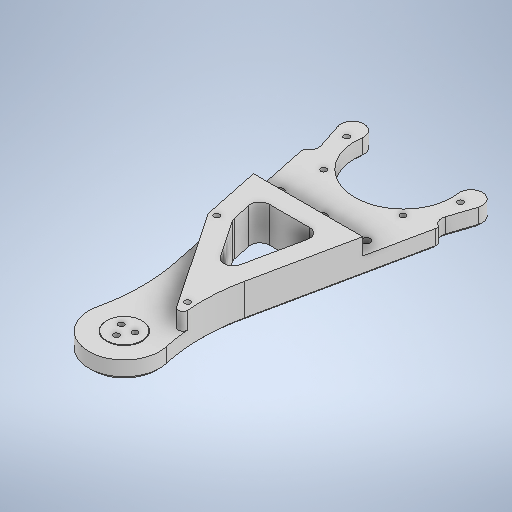
# Autodesk Inventor part: motion_thigh_top_R
Saved by Autodesk Inventor 2025.2 (Build 292293000, 293)
## iProperties
Created: 2025-04-10
Part Number: motion_thigh_top_R
Material: Generic
Document SubType Name: Modeling
Designer: Bruno
Density: 1 g/cm^3
Appearance: Default
Mass: 96.8952 g
Surface Area: 228.709 cm^2
Volume: 96.8952 cm^3
Author: Bruno
## iProperties of the stored document motion_thigh_top_R_3DPrint.ipt
Created: 2025-04-29
Part Number: motion_thigh_top_R_3DPrint
Material: Generic
Document SubType Name: Modeling
Designer: Bruno
Density: 1 g/cm^3
Appearance: Default
Author: Bruno
Autodesk Inventor part; units mm, degrees
ref_plane "YZ Plane" through (0, 0, 0) normal (1, 0, 0) x (0, 1, 0)
ref_plane "XZ Plane" through (0, 0, 0) normal (0, 1, 0) x (-1, 0, 0)
ref_plane "XY Plane" through (0, 0, 0) normal (0, 0, 1) x (1, 0, 0)
sketch "Sketch1" plane through (0, 0, 0) normal (0, 1, 0) x (-1, 0, 0)
  line L0 (0, -140.06) -> (0, 133.01) construction
  line L1 (42.5247, -92.2999) -> (20, -23.7432)
  line L2 (20, -23.7432) -> (-20, -23.7432) construction
  line L3 (-20, -23.7432) -> (-42.5247, -92.2999)
  circle A0 centre (30.55, -75) radius 1.5
  circle A1 centre (21.275, -53.4355) radius 1.5
  circle A2 centre (12, -31.8711) radius 2
  circle A3 centre (0, -31.8711) radius 2
  circle A4 centre (-12, -31.8711) radius 2
  circle A5 centre (-21.275, -53.4355) radius 1.5
  circle A6 centre (-30.55, -75) radius 1.5
  circle A7 centre (0, -75) radius 26.05
  line L4 (0, -75) -> (0, 75) construction
  arc A8 (18.259, 69.7455) -> (-18.259, 69.7455) centre (0, 75) ccw
  arc A9 (18.259, 69.7455) -> (20, -23.7432) centre (170.8734, 25.8271) ccw
  arc A10 (-20, -23.7432) -> (-18.259, 69.7455) centre (-170.8734, 25.8271) ccw
  circle A11 centre (31.8586, -79.425) radius 6.1144
  circle A12 centre (-31.8586, -79.425) radius 6.1144
  point P0 (0, 0)
  point P1 (37.6675, -77.5164)
  point P2 (-37.6675, -77.5164)
  point P3 (-25.8023, -78.5838)
  point P4 (25.8023, -78.5838)
  dimension "d0" = 3
  dimension "d1" = 52.1
  dimension "d2" = 4
  dimension "d3" = 36.376
  dimension "d4" = 108.188
  dimension "d5" = 80.8
  dimension "d6" = 68.5567
  dimension "d7" = 80.8
  dimension "d8" = 5.9764
  dimension "d9" = 64.0236
  dimension "d10" = 35
  dimension "d11" = 35
  dimension "d12" = 64.0236
  dimension "d13" = 5.9764
  dimension "d14" = 8.0569
  dimension "d15" = 48.4809
  dimension "d16" = 48.4809
  dimension "d17" = 8.0569
  dimension "d18" = 10.1373
  dimension "d19" = 32.9382
  dimension "d20" = 21.5378
  dimension "d21" = 21.5378
  dimension "d22" = 32.9382
  dimension "d23" = 10.1373
  dimension "d24" = 150
  dimension "d25" = 38
  dimension "d26" = 75
  constraints: 13 centre point, 10 tangent, 8 end point, 6 point on circle, 5 equal radius, 2 point on line, 2 vertical alignment, 1 coincident
  measures "d0" diameter of A0
  measures "d1" diameter of A7
  measures "d2" diameter of A2
  measures "d3" angle of L1 L3
  measures "d4" angle of L1 L2
  measures "d5" distance from line of L1.start L3
  measures "d6" distance from line of L1.start L2
  measures "d7" distance from line of L3.end L1
  measures "d8" distance from line of A0.centre L1
  measures "d9" distance from line of A0.centre L3
  measures "d10" distance from line of L4.start L1
  measures "d11" distance from line of L4.start L3
  measures "d12" distance from line of A6.centre L1
  measures "d13" distance from line of A6.centre L3
  measures "d14" distance from line of A1.centre L1
  measures "d15" distance from line of A1.centre L3
  measures "d16" distance from line of A5.centre L1
  measures "d17" distance from line of A5.centre L3
  measures "d18" distance from line of A2.centre L1
  measures "d19" distance from line of A2.centre L3
  measures "d20" distance from line of A3.centre L1
  measures "d21" distance from line of A3.centre L3
  measures "d22" distance from line of A4.centre L1
  measures "d23" distance from line of A4.centre L3
  measures "d24" distance of L4.start L4.end
  measures "d25" diameter of A8
  measures "d26" distance of point (0, 0) L4.end
extrude "Extrusion1" add sketch "Sketch1" along normal blind 10 contours A11 A7 A12 L3 A10 A8 A9 L1 | A11 | A12 | A2 | A4
sketch "Sketch2" plane through (0, 0, 0) normal (0, -1, 0) x (1, 0, 0)
  arc A0 (18.259, 69.7455) -> (20, -23.7432) centre (170.8734, 25.8271) ccw projected
  line L0 (20, -23.7432) -> (-20, -23.7432)
  arc A1 (18.259, 69.7455) -> (-18.259, 69.7455) centre (0, 75) ccw projected
  arc A2 (-20, -23.7432) -> (-18.259, 69.7455) centre (-170.8734, 25.8271) ccw projected
  circle A3 centre (0, 75) radius 24 construction
  arc A4 (-8.448, 56.1313) -> (-14.4134, 53.0348) centre (-10.9405, 53.6387) ccw
  arc A5 (12.2645, 33.7778) -> (11.2365, 36.4468) centre (8.7439, 33.9542) ccw
  line L1 (-8.448, 56.1313) -> (11.2365, 36.4468)
  line L2 (0, 75) -> (0, 70.3396) construction
  point P0 (0, 0)
  dimension "d30" = 48
  dimension "d31" = 7.05
  dimension "d32" = 7.05
  dimension "d33" = 45
  constraints: 6 end point, 6 point on circle, 4 tangent, 2 centre point, 1 coincident, 1 vertical, 3 other
  measures "d31" diameter of A4
  measures "d32" diameter of A5
  measures "d33" angle of L1 L2
sketch "Sketch4" plane through (0, 10, 0) normal (0, 1, 0) x (1, 0, 0)
  arc A0 (-18.259, -69.7455) -> (18.259, -69.7455) centre (0, -75) ccw projected
  circle A1 centre (0, -75) radius 8.5 construction
  line L0 (-3.6806, -70.075) -> (3.6806, -70.075) construction
  line L1 (2.4249, -80.65) -> (6.1055, -74.275) construction
  line L2 (-2.4249, -80.65) -> (-6.1055, -74.275) construction
  circle A2 centre (0, -75) radius 4.25 construction
  arc A3 (-2.7639, -79.6984) -> (2.7639, -79.6984) centre (0, -79.25) ccw
  arc A4 (5.4509, -75.0444) -> (2.687, -70.2572) centre (3.6806, -72.875) ccw
  arc A5 (-2.687, -70.2572) -> (-5.4509, -75.0444) centre (-3.6806, -72.875) ccw
  arc A6 (-2.687, -70.2572) -> (2.687, -70.2572) centre (0, -63.1778) ccw
  arc A7 (-2.7639, -79.6984) -> (-5.4509, -75.0444) centre (-10.2383, -80.9111) ccw
  arc A8 (5.4509, -75.0444) -> (2.7639, -79.6984) centre (10.2383, -80.9111) ccw
  point P0 (0, 0)
  dimension "d40" = 17
  dimension "d46" = 2.8
  dimension "d47" = 2.8
  dimension "d48" = 2.8
  dimension "d50" = 8.5
  constraints: 21 point on circle, 13 tangent, 8 centre point, 6 end point, 2 coincident, 2 equal length, 2 equal radius, 1 horizontal
  measures "d40" diameter of A1
  measures "d46" radius of A5
  measures "d47" radius of A4
  measures "d48" radius of A3
  measures "d50" diameter of A2
extrude "Extrusion4" cut sketch "Sketch4" against normal blind 3
sketch "Sketch5" plane through (0, 7, 0) normal (0, 1, 0) x (1, 0, 0)
  arc A0 (-2.687, -70.2572) -> (-5.4509, -75.0444) centre (-3.6806, -72.875) ccw projected
  circle A1 centre (-3.6806, -72.875) radius 1.5
  arc A2 (5.4509, -75.0444) -> (2.687, -70.2572) centre (3.6806, -72.875) ccw projected
  circle A3 centre (3.6806, -72.875) radius 1.5
  arc A4 (-2.7639, -79.6984) -> (2.7639, -79.6984) centre (0, -79.25) ccw projected
  circle A5 centre (0, -79.25) radius 1.5
  point P0 (0, 0)
  point P1 (-6.1055, -74.275)
  point P2 (-3.6806, -70.075)
  point P3 (3.6806, -70.075)
  point P4 (6.1055, -74.275)
  point P5 (2.4249, -80.65)
  point P6 (-2.4249, -80.65)
  dimension "d53" = 3
  dimension "d54" = 3
  dimension "d55" = 3
  constraints: 3 centre point, 3 coincident
  measures "d53" diameter of A1
  measures "d54" diameter of A5
  measures "d55" diameter of A3
extrude "Extrusion5" cut sketch "Sketch5" against normal through all
sketch "Sketch10" plane through (0, 10, 0) normal (0, 1, 0) x (1, 0, 0)
  point P0 (0, 0)
sketch "Sketch11" plane through (0, 10, 0) normal (0, 1, 0) x (1, 0, 0)
  circle A0 centre (23.2705, 31.8711) radius 2 projected
  circle A1 centre (-23.2705, 31.8711) radius 2 projected
  arc A2 (36.124, 56.2492) -> (35.2621, 58.3316) centre (34.1663, 56.6585) ccw projected
  arc A3 (33.2513, 64.0751) -> (35.2621, 58.3316) centre (38.0015, 62.5144) ccw projected
  line L0 (33.2513, 64.0751) -> (42.5247, 92.2999) projected
  arc A4 (37.4868, 95.4546) -> (42.5247, 92.2999) centre (43.0738, 98.7767) ccw projected
  line L1 (13.5182, 103.3296) -> (37.4868, 95.4546) projected
  line L2 (13.5182, 103.3296) -> (21.946, 128.9806) projected
  line L3 (44.7468, 121.4892) -> (21.946, 128.9806) projected
  line L4 (44.7468, 121.4892) -> (45.9436, 125.1317) projected
  arc A5 (45.9436, 125.1317) -> (-45.9436, 125.1317) centre (0, 75) ccw projected
  line L5 (-45.9436, 125.1317) -> (-41.8595, 112.7014) projected
  line L6 (-41.8595, 112.7014) -> (-19.0587, 120.1928) projected
  line L7 (-19.0587, 120.1928) -> (-16.4055, 112.1174) projected
  line L8 (-16.4055, 112.1174) -> (-39.2064, 104.6261) projected
  line L9 (-39.2064, 104.6261) -> (-38.9298, 103.7845) projected
  arc A6 (-42.5247, 92.2999) -> (-38.9298, 103.7845) centre (-43.0738, 98.7767) ccw projected
  line L10 (-42.5247, 92.2999) -> (-33.2513, 64.0751) projected
  arc A7 (-35.2621, 58.3316) -> (-33.2513, 64.0751) centre (-38.0015, 62.5144) ccw projected
  arc A8 (-35.2621, 58.3316) -> (-36.124, 56.2492) centre (-34.1663, 56.6585) ccw projected
  line L11 (-36.124, 56.2492) -> (-29.328, 23.7432) projected
  line L12 (-29.328, 23.7432) -> (29.328, 23.7432) projected
  line L13 (29.328, 23.7432) -> (36.124, 56.2492) projected
  circle A9 centre (-30.55, 75) radius 1.5 projected
  circle A10 centre (0, 31.8711) radius 2 projected
  circle A11 centre (30.55, 75) radius 1.5 projected
  circle A12 centre (-21.275, 53.4355) radius 1.5 projected
  circle A13 centre (21.275, 53.4355) radius 1.5 projected
  circle A14 centre (0, 75) radius 26.05 projected
  line L14 (-8.6089, 110.8133) -> (-15.4999, 131.7869) projected
  arc A15 (-14.0608, 134.3573) -> (-15.4999, 131.7869) centre (-13.5998, 132.4112) ccw projected
  arc A16 (14.0608, 134.3573) -> (-14.0608, 134.3573) centre (0, 75) ccw projected
  arc A17 (15.4999, 131.7869) -> (14.0608, 134.3573) centre (13.5998, 132.4112) ccw projected
  line L15 (15.4999, 131.7869) -> (8.6089, 110.8133) projected
  arc A18 (6.3466, 109.4706) -> (8.6089, 110.8133) centre (6.7088, 111.4375) ccw projected
  arc A19 (6.3466, 109.4706) -> (-6.3466, 109.4706) centre (0, 75) ccw projected
  arc A20 (-8.6089, 110.8133) -> (-6.3466, 109.4706) centre (-6.7088, 111.4375) ccw projected
  line L16 (20, 23.7432) -> (37.6675, 77.5164) projected
  line L17 (-37.6675, 77.5164) -> (-20, 23.7432) projected
  point P0 (0, 0)
  point P1 (22.1305, 30.2277)
  point P2 (23.3273, 33.8703)
  point P3 (-23.3273, 33.8703)
  point P4 (-22.1305, 30.2277)
extrude "Extrusion8" add sketch "Sketch11" against normal up to surface (10 mm away) contours A0 L16 | A0 L16 A3 A2 L13 L12 | L16 A0 | L12 L11 A8 A7 L17 A1 | L17 A1 | A1 L17
sketch "Sketch12" plane through (0, 10, 0) normal (0, 1, 0) x (1, 0, 0)
  circle A0 centre (-23.2705, 31.8711) radius 2 projected
  circle A1 centre (23.2705, 31.8711) radius 2 projected
  point P0 (0, 0)
extrude "Extrusion9" cut sketch "Sketch12" against normal through all
sketch "Sketch13" plane through (0, 10, 0) normal (0, 1, 0) x (1, 0, 0)
  line L0 (-36.124, 56.2492) -> (-29.328, 23.7432) projected
  line L1 (-29.328, 23.7432) -> (-18.3221, -28.899)
  arc A0 (-18.259, -69.7455) -> (18.259, -69.7455) centre (0, -75) ccw projected
  circle A1 centre (0, -75) radius 19
  arc A2 (-18.5539, -70.9068) -> (-18.3221, -28.899) centre (-116.2057, -49.3635) ccw
  line L2 (0, -56) -> (0, -94) construction
  line L3 (29.328, 23.7432) -> (18.3221, -28.899)
  arc A3 (18.3221, -28.899) -> (18.5539, -70.9068) centre (116.2057, -49.3635) ccw
  arc A4 (-18.259, -69.7455) -> (-20, 23.7432) centre (-170.8734, -25.8271) ccw projected
  line L4 (-29.328, 23.7432) -> (-20, 23.7432) projected
  line L5 (20, 23.7432) -> (29.328, 23.7432) projected
  arc A5 (20, 23.7432) -> (18.259, -69.7455) centre (170.8734, -25.8271) ccw projected
  point P0 (0, 0)
  point P1 (0, -75)
  point P2 (18.5539, -70.9068)
  point P3 (-18.5539, -70.9068)
  dimension "d67" = 100
  constraints: 8 point on circle, 6 end point, 4 symmetric about line, 3 centre point, 2 tangent, 1 coincident, 1 collinear, 1 concentric, 1 midpoint, 1 vertical alignment, 1 other
  measures "d67" radius of A2
extrude "Extrusion10" add sketch "Sketch13" against normal up to surface (10 mm away) contours L4 A4 A0 A2 L1 | A5 L5 L3 A3 A0
chamfer "Chamfer1" distance 2 angle 45 14 edges at (-27.2231, 10, -13.6751) (-16.2072, 10, 49.9152) (0, 10, 94) (16.2072, 10, 49.9152) (27.2231, 10, -13.6751) (36.0143, 10, -57.4234) (33.2823, 10, -60.8622) (35.4594, 10, -70.7958) (32.4064, 10, -85.5148) (0, 10, -48.95) (-32.4064, 10, -85.5148) (-35.4594, 10, -70.7958) (-33.2823, 10, -60.8622) (-36.0143, 10, -57.4234)
sketch "Sketch24" plane through (0, 0, 0) normal (0, -1, 0) x (1, 0, 0)
  line L0 (4.2583, 47.3257) -> (-95.4066, -100.5193) projected
  line L1 (-29.328, -23.7432) -> (29.328, -23.7432) projected
  arc A0 (18.5539, 70.9068) -> (18.3221, 28.899) centre (116.2057, 49.3635) ccw projected
  circle A1 centre (-23.2705, -31.8711) radius 2 projected
  circle A2 centre (23.2705, -31.8711) radius 2 projected
  arc A3 (18.5539, 70.9068) -> (-18.5539, 70.9068) centre (0, 75) ccw projected
  arc A4 (-18.3221, 28.899) -> (-18.5539, 70.9068) centre (-116.2057, 49.3635) ccw projected
  line L2 (-18.3221, 28.899) -> (-36.124, -56.2492) projected
  arc A5 (-36.124, -56.2492) -> (-35.2621, -58.3316) centre (-34.1663, -56.6585) ccw projected
  arc A6 (-33.2513, -64.0751) -> (-35.2621, -58.3316) centre (-38.0015, -62.5144) ccw projected
  line L3 (-37.6675, -77.5164) -> (-33.2513, -64.0751) projected
  arc A7 (-37.6675, -77.5164) -> (-25.8023, -78.5838) centre (-31.8586, -79.425) ccw projected
  arc A8 (25.8023, -78.5838) -> (-25.8023, -78.5838) centre (0, -75) ccw projected
  arc A9 (25.8023, -78.5838) -> (37.6675, -77.5164) centre (31.8586, -79.425) ccw projected
  line L4 (33.2513, -64.0751) -> (37.6675, -77.5164) projected
  arc A10 (35.2621, -58.3316) -> (33.2513, -64.0751) centre (38.0015, -62.5144) ccw projected
  arc A11 (35.2621, -58.3316) -> (36.124, -56.2492) centre (34.1663, -56.6585) ccw projected
  line L5 (36.124, -56.2492) -> (18.3221, 28.899) projected
  arc A12 (18.5539, 70.9068) -> (18.3221, 28.899) centre (116.2057, 49.3635) ccw projected
  circle A13 centre (3.6806, 72.875) radius 1.5 projected
  circle A14 centre (0, 79.25) radius 1.5 projected
  circle A15 centre (-3.6806, 72.875) radius 1.5 projected
  circle A16 centre (-30.55, -75) radius 1.5 projected
  circle A17 centre (30.55, -75) radius 1.5 projected
  circle A18 centre (0, -31.8711) radius 2 projected
  circle A19 centre (21.275, -53.4355) radius 1.5 projected
  circle A20 centre (-21.275, -53.4355) radius 1.5 projected
  line L6 (4.2583, 47.3257) -> (17.8664, 67.5123)
  point P0 (0, 0)
  point P1 (-22.8891, 7.0548)
  point P2 (18.3221, 28.899)
  constraints: 2 end point, 1 collinear, 1 point on circle
extrude "Extrusion20" add sketch "Sketch24" along normal blind 9 contours L6 A0 L5 L1 L2 L0
sketch "Sketch25" plane through (0, -9, 0) normal (0, -1, 0) x (1, 0, 0)
  circle A0 centre (13.8445, 83.053) radius 1.5 projected
  circle A1 centre (-8.053, 88.8445) radius 1.5 projected
  circle A2 centre (8.053, 61.1555) radius 1.5 projected
  circle A3 centre (-13.8445, 66.947) radius 1.5 projected
  circle A4 centre (57.0388, 59.9143) radius 1.5 projected
  circle A5 centre (0, 75) radius 12.1825 projected
  line L0 (54.7376, 51.2135) -> (22.5353, 59.7304) projected
  arc A6 (54.7376, 51.2135) -> (59.34, 68.6151) centre (57.0388, 59.9143) ccw projected
  line L1 (27.1377, 77.132) -> (59.34, 68.6151) projected
  arc A7 (15.9979, 85.2502) -> (27.1377, 77.132) centre (31.9958, 95.5005) ccw projected
  arc A8 (15.9979, 85.2502) -> (8.8386, 58.181) centre (0, 75) ccw projected
  arc A9 (22.5353, 59.7304) -> (8.8386, 58.181) centre (17.6772, 41.362) ccw projected
  line L2 (17.8664, 67.5123) -> (-22.8891, 7.0548) projected
  line L3 (-22.8891, 7.0548) -> (-29.328, -23.7432) projected
  line L4 (-29.328, -23.7432) -> (29.328, -23.7432) projected
  line L5 (29.328, -23.7432) -> (18.3221, 28.899) projected
  arc A10 (17.8664, 67.5123) -> (18.3221, 28.899) centre (116.2057, 49.3635) ccw projected
  circle A11 centre (14.0822, 57.5183) radius 2.4486
  arc A12 (17.8664, 67.5123) -> (18.3221, 28.899) centre (116.2057, 49.3635) ccw projected
  arc A13 (-22.5029, 7.6276) -> (-23.0304, 6.3786) centre (-19.58, 5.6572) ccw
  point P0 (0, 0)
  point P1 (16.523, 57.3234)
  point P2 (12.0519, 58.8869)
  dimension "d117" = 7.05
  constraints: 5 tangent, 2 centre point, 2 point on circle, 2 point on line
  measures "d117" diameter of A13
extrude "Extrusion21" cut sketch "Sketch25" against normal up to surface (9 mm away) contours A10 A11 A9 | A9 L2 A10 | A11 L2 A9 | A13 L3 L2
sketch "Sketch26" plane through (0, -9, 0) normal (0, -1, 0) x (1, 0, 0)
  circle A0 centre (12.7693, 53.6449) radius 3.525 construction
  arc A1 (16.523, 57.3234) -> (18.3221, 28.899) centre (116.2057, 49.3635) ccw projected
  line L0 (12.0519, 58.8869) -> (-22.5029, 7.6276) projected
  circle A2 centre (12.7693, 53.6449) radius 1.5
  arc A3 (-22.5029, 7.6276) -> (-23.0304, 6.3786) centre (-19.58, 5.6572) ccw projected
  circle A4 centre (-19.58, 5.6572) radius 1.5
  point P0 (0, 0)
  dimension "d120" = 7.05
  dimension "d121" = 3
  dimension "d122" = 3
  constraints: 3 centre point, 2 coincident, 2 tangent
  measures "d120" diameter of A0
  measures "d121" diameter of A2
  measures "d122" diameter of A4
extrude "Extrusion22" cut sketch "Sketch26" against normal through all
sketch "Sketch27" plane through (0, 10, 0) normal (0, 1, 0) x (1, 0, 0)
  circle A0 centre (-19.58, -5.6572) radius 1.5 projected
  circle A1 centre (-19.58, -5.6572) radius 2.8
  circle A2 centre (12.7693, -53.6449) radius 1.5 projected
  circle A3 centre (12.7693, -53.6449) radius 2.8
  point P0 (0, 0)
  dimension "d125" = 5.6
  dimension "d126" = 5.6
  constraints: 2 centre point, 2 coincident
  measures "d125" diameter of A1
  measures "d126" diameter of A3
extrude "Extrusion23" cut sketch "Sketch27" against normal blind 3 contours A0 | A1 | A2 | A3
sketch "Sketch28" plane through (0, -9, 0) normal (0, -1, 0) x (1, 0, 0)
  circle A0 centre (-19.58, 5.6572) radius 1.5 projected
  circle A1 centre (12.7693, 53.6449) radius 1.5 projected
  arc A2 (-22.5029, 7.6276) -> (-23.0304, 6.3786) centre (-19.58, 5.6572) ccw projected
  line L0 (-23.0304, 6.3786) -> (-29.328, -23.7432) projected
  line L1 (-29.328, -23.7432) -> (29.328, -23.7432) projected
  line L2 (29.328, -23.7432) -> (18.3221, 28.899) projected
  arc A3 (16.523, 57.3234) -> (18.3221, 28.899) centre (116.2057, 49.3635) ccw projected
  arc A4 (16.523, 57.3234) -> (12.0519, 58.8869) centre (14.0822, 57.5183) ccw projected
  line L3 (12.0519, 58.8869) -> (-22.5029, 7.6276) projected
  line L4 (-13.5018, 3.0901) -> (-17.0211, -13.7432)
  line L5 (-17.0211, -13.7432) -> (17.0211, -13.7432)
  line L6 (17.0211, -13.7432) -> (8.5337, 26.8526)
  arc A5 (7.2928, 33.9371) -> (8.5337, 26.8526) centre (116.2057, 49.3635) ccw
  line L7 (7.2928, 33.9371) -> (-13.5018, 3.0901)
  point P0 (0, 0)
  dimension "d129" = 10
  constraints: 8 end point, 2 point on circle, 1 centre point, 4 other
  measures "d129" distance between parallel lines of L3 L7
extrude "Extrusion24" cut sketch "Sketch28" against normal through all contours L7 A5 L6 L5 L4
fillet "Fillet2" radius 5 4 edges at (7.2928, 0.5, 33.9371) (17.0211, 0.5, -13.7432) (-13.5018, 0.5, 3.0901) (-17.0211, 0.5, -13.7432)
mirror "Mirror1" about plane through (0, 0, 0) normal (0, 1, 0) remove original yes
sketch "Sketch29" plane through (0, -10, -75) normal (0, -1, 0) x (1, 0, 0)
  circle A0 centre (30.55, 0) radius 1.5 projected
  circle A1 centre (30.55, 0) radius 2.8
  circle A2 centre (21.275, 21.5645) radius 1.5 projected
  circle A3 centre (21.275, 21.5645) radius 2.8
  circle A4 centre (-21.275, 21.5645) radius 1.5 projected
  circle A5 centre (-21.275, 21.5645) radius 2.8
  circle A6 centre (-30.55, 0) radius 1.5 projected
  circle A7 centre (-30.55, 0) radius 2.8
  point P0 (0, 75)
  dimension "d133" = 5.6
  dimension "d134" = 5.6
  dimension "d135" = 5.6
  dimension "d136" = 5.6
  constraints: 4 centre point, 4 coincident
  measures "d133" diameter of A1
  measures "d134" diameter of A3
  measures "d135" diameter of A5
  measures "d136" diameter of A7
extrude "Extrusion25" cut sketch "Sketch29" against normal blind 3 contours A0 | A1 | A3 | A4 | A5 | A6 | A7
sketch "Sketch30" plane through (0, -7, 75) normal (0, -1, 0) x (1, 0, 0)
  circle A0 centre (3.6806, -2.125) radius 1.5 projected
  circle A1 centre (0, 4.25) radius 1.5 projected
  circle A2 centre (-3.6806, -2.125) radius 1.5 projected
  arc A3 (2.7639, 4.6984) -> (5.4509, 0.0444) centre (10.2383, 5.9111) ccw projected
  arc A4 (2.7639, 4.6984) -> (-2.7639, 4.6984) centre (0, 4.25) ccw projected
  arc A5 (-5.4509, 0.0444) -> (-2.7639, 4.6984) centre (-10.2383, 5.9111) ccw projected
  arc A6 (-5.4509, 0.0444) -> (-2.687, -4.7428) centre (-3.6806, -2.125) ccw projected
  arc A7 (2.687, -4.7428) -> (-2.687, -4.7428) centre (0, -11.8222) ccw projected
  arc A8 (2.687, -4.7428) -> (5.4509, 0.0444) centre (3.6806, -2.125) ccw projected
  line L0 (2.3643, 5.75) -> (-2.3643, 5.75)
  line L1 (3.3575, 2.75) -> (-3.3575, 2.75)
  line L2 (6.0449, -0.625) -> (-6.0449, -0.625)
  line L3 (-6.0449, -3.625) -> (6.0449, -3.625)
  point P0 (0, -75)
  constraints: 8 end point, 8 point on circle, 4 tangent, 3 parallel, 1 horizontal
extrude "Extrusion26" add sketch "Sketch30" along normal blind 0.2 contours L2 A6 A5 L1 A3 A8 | L3 A8 A7 A6 | L0 A4
sketch "Sketch31" plane through (12.7693, -7, 53.6449) normal (0, -1, 0) x (1, 0, 0)
  circle A0 centre (0, 0) radius 1.5 projected
  circle A1 centre (0, 0) radius 2.8 projected
  circle A2 centre (-32.3493, -47.9877) radius 1.5 projected
  circle A3 centre (-32.3493, -47.9877) radius 2.8 projected
  circle A4 centre (-34.0443, -107.0804) radius 1.5 projected
  circle A5 centre (-34.0443, -107.0804) radius 2.8 projected
  circle A6 centre (8.5057, -107.0804) radius 2.8 projected
  circle A7 centre (8.5057, -107.0804) radius 1.5 projected
  circle A8 centre (17.7807, -128.6449) radius 1.5 projected
  circle A9 centre (17.7807, -128.6449) radius 2.8 projected
  line L0 (2.3643, 1.5) -> (-2.3643, 1.5)
  line L1 (2.3643, -1.5) -> (-2.4597, -1.5)
  line L2 (-29.985, -46.4877) -> (-34.7136, -46.4877)
  line L3 (-29.985, -49.4877) -> (-34.7136, -49.4877)
  circle A10 centre (-32.3493, -47.9877) radius 1.5 projected
  line L4 (-31.68, -105.5804) -> (-36.4086, -105.5804)
  line L5 (-31.68, -108.5804) -> (-36.4086, -108.5804)
  circle A11 centre (-34.0443, -107.0804) radius 1.5 projected
  circle A12 centre (-43.3193, -128.6449) radius 1.5 projected
  circle A13 centre (-43.3193, -128.6449) radius 2.8 projected
  line L6 (-40.955, -127.1449) -> (-45.6836, -127.1449)
  line L7 (-40.955, -130.1449) -> (-45.6836, -130.1449)
  circle A14 centre (-43.3193, -128.6449) radius 1.5 projected
  line L8 (10.87, -105.5804) -> (6.1414, -105.5804)
  line L9 (10.87, -108.5804) -> (6.1414, -108.5804)
  circle A15 centre (8.5057, -107.0804) radius 1.5 projected
  line L10 (20.145, -127.1449) -> (15.4164, -127.1449)
  line L11 (20.145, -130.1449) -> (15.4164, -130.1449)
  point P0 (-12.7693, -53.6449)
  point P1 (-2.3643, -1.5)
  constraints: 24 end point, 23 point on circle, 12 tangent, 7 horizontal, 5 parallel
extrude "Extrusion27" add sketch "Sketch31" along normal blind 0.2 contours L0 A1 | L1 A1 | L2 A3 | L3 A3 | L4 A5 | L5 A5 | L8 A6 | A6 L9 | L10 A9 | L11 A9 | L6 A13 | L7 A13
fillet "Fillet3" radius 0.4 8 edges at (15.0703, -9.1711, 52.0495) (15.1535, -9.2156, 55.113) (-22.3208, -8.725, 6.2302) (19.3085, -9.4428, -55.4288) (27.75, -9.7, -75) (-19.3085, -9.4428, -55.4288) (-27.8308, -9.7888, -75.6678) (-27.8309, -9.7889, -74.3319)
sketch "Sketch32" plane through (0, 0, 75) normal (0, 1, 0) x (1, 0, 0)
  line L0 (-22.5029, 67.3724) -> (12.0519, 16.1131) projected
  arc A0 (-23.0304, 68.6214) -> (-22.5029, 67.3724) centre (-19.58, 69.3428) ccw projected
  line L1 (-18.3221, 46.101) -> (-23.0304, 68.6214) projected
  arc A1 (-18.5539, 4.0932) -> (-18.3221, 46.101) centre (-116.2057, 25.6365) ccw projected
  arc A2 (-18.5539, 4.0932) -> (18.5539, 4.0932) centre (0, 0) ccw projected
  arc A3 (16.523, 17.6766) -> (18.5539, 4.0932) centre (116.2057, 25.6365) ccw projected
  arc A4 (12.0519, 16.1131) -> (16.523, 17.6766) centre (14.0822, 17.4817) ccw projected
  circle A5 centre (3.6806, 2.125) radius 1.5 projected
  circle A6 centre (0, -4.25) radius 1.5 projected
  circle A7 centre (-3.6806, 2.125) radius 1.5 projected
  circle A8 centre (0, 0) radius 8.5 construction
  circle A9 centre (0, 0) radius 9.35
  point P0 (0, 75)
  dimension "d144" = 17
  dimension "d145" = 0.85
  constraints: 2 centre point, 2 coincident
  measures "d144" diameter of A8
  measures "d145" radial gap between concentric circles of A9 A8
extrude "Extrusion28" cut sketch "Sketch32" against normal blind 0.2 contours L0 A4 A3 A2 A1 L1 A0
chamfer "Chamfer2" distance 0.2 angle 45 1 edges at (-9.35, -0.2, 75)
equation "\"d26\" = 0.5 * d24"
body "Solid1"
